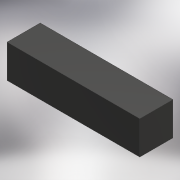
# Autodesk Inventor part: 1420-06 Meuble noir
Saved by Autodesk Inventor 2017 (Build 210142000, 142)
## iProperties
Part Number: 1420-06 Meuble noir
Project: 1420 VAUBAN 3D XL
Material: Bois (bouleau)
Catalog Web Link: http://www.frenchmakers.com/
Document SubType Name: Modeling
Designer: Adrien MARY
Mass: 275000 g
Surface Area: 45000 cm^2
Volume: 500000 cm^3
Density: 0.55 g/cm^3
Appearance: Lisse - Noir
Company: FABLAB Frenchmakers
Author: Adrien MARY
Autodesk Inventor part; units mm, degrees
ref_plane "YZ Plane" through (0, 0, 0) normal (1, 0, 0) x (0, 1, 0)
ref_plane "XZ Plane" through (0, 0, 0) normal (0, 1, 0) x (-1, 0, 0)
ref_plane "XY Plane" through (0, 0, 0) normal (0, 0, 1) x (1, 0, 0)
sketch "Esquisse1" plane through (0, 0, 0) normal (0, 0, 1) x (1, 0, 0)
  line L0 (-1000, -250) -> (1000, -250)
  line L1 (1000, -250) -> (1000, 250)
  line L2 (1000, 250) -> (-1000, 250)
  line L3 (-1000, 250) -> (-1000, -250)
  line L4 (-1000, -250) -> (1000, 250) construction
  line L5 (1000, -250) -> (-1000, 250) construction
  point P0 (0, 0)
  dimension "d0" = 2000
  dimension "d1" = 500
  constraints: 12 end point, 2 midpoint, 2 parallel, 1 horizontal, 1 perpendicular
  measures "d0" distance of L2.end L1.end
  measures "d1" distance of L1.end L0.end
extrude "Extrusion1" add sketch "Esquisse1" along normal blind 500
